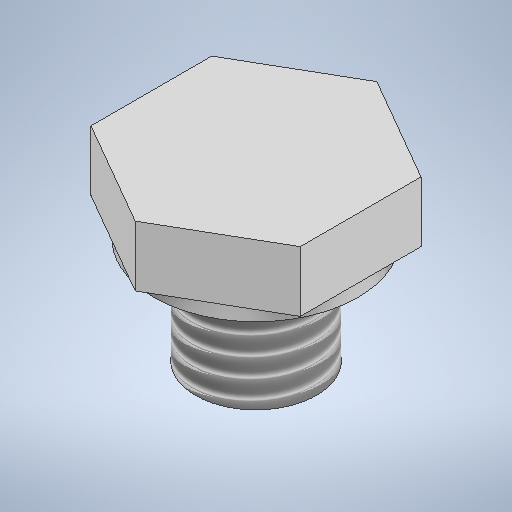
# Autodesk Inventor part: 123 cap
Saved by Autodesk Inventor 2025.1 (Build 291241000, 241)
## iProperties
Created: 2024-08-21
Part Number: 123 cap
Material: Generisch
Document SubType Name: Modeling
Designer: ffogue
Density: 1 g/cm^3
Appearance: Vorgabe
Author: ffogue
Autodesk Inventor part; units mm, degrees
ref_plane "YZ Plane" through (0, 0, 0) normal (1, 0, 0) x (0, 1, 0)
ref_plane "XZ Plane" through (0, 0, 0) normal (0, 1, 0) x (-1, 0, 0)
ref_plane "XY Plane" through (0, 0, 0) normal (0, 0, 1) x (1, 0, 0)
sketch "Sketch1" plane through (0, 0, 0) normal (0, 0, 1) x (1, 0, 0)
  line L0 (0, 8) -> (6.9282, 4)
  line L1 (6.9282, 4) -> (6.9282, -4)
  line L2 (6.9282, -4) -> (0, -8)
  line L3 (0, -8) -> (-6.9282, -4)
  line L4 (-6.9282, -4) -> (-6.9282, 4)
  line L5 (-6.9282, 4) -> (0, 8)
  point P0 (0, 0)
  point P1 (0, 0)
  point P2 (-6.9282, 0)
  dimension "d0" = 16
  constraints: 12 end point, 1 coincident, 1 horizontal alignment, 1 midpoint, 13 other
  measures "d0" distance of L2.end L0.start
extrude "Extrusion1" add sketch "Sketch1" along normal blind 4
sketch "Sketch2" plane through (0, 0, 0) normal (0, 0, -1) x (-1, 0, 0)
  circle A0 centre (0, 0) radius 4
  dimension "d3" = 8
  constraints: 1 centre point, 1 coincident
  measures "d3" diameter of A0
extrude "Extrusion2" add sketch "Sketch2" along normal blind 8
sketch "Sketch3" plane through (0, 0, 0) normal (0, 0, -1) x (-1, 0, 0)
  circle A0 centre (0, 0) radius 6.75
  circle A1 centre (0, 0) radius 4
  dimension "d6" = 13.5
  dimension "d7" = 8
  constraints: 2 centre point, 2 coincident
  measures "d6" diameter of A0
  measures "d7" diameter of A1
extrude "Extrusion3" add sketch "Sketch3" along normal blind 1 separate body
thread "Thread1" size "M8x1.25" class "6g" standard "ISO Metric profile" length 7
body "Solid1"
